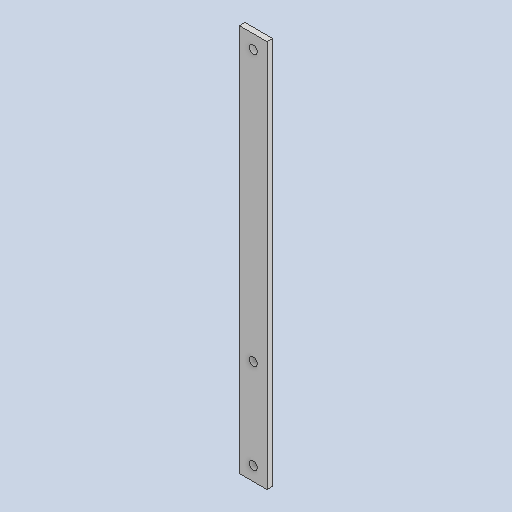
# Autodesk Inventor part: レール接続
Saved by Autodesk Inventor 2022 (Build 260153070, 153G)
## iProperties
Created: 2022-10-17
Part Number: レール接続
Material: 一般
Document SubType Name: Modeling
Designer: hirok
Density: 1 g/cm^3
Appearance: 既定
Author: hirok
Autodesk Inventor part; units mm, degrees
ref_plane "YZ Plane" through (0, 0, 0) normal (1, 0, 0) x (0, 1, 0)
ref_plane "XZ Plane" through (0, 0, 0) normal (0, 1, 0) x (-1, 0, 0)
ref_plane "XY Plane" through (0, 0, 0) normal (0, 0, 1) x (1, 0, 0)
sketch "スケッチ1" plane through (0, 0, 0) normal (0, 0, 1) x (1, 0, 0)
  line L0 (0, 0) -> (10, 0)
  line L1 (10, 0) -> (10, 140)
  line L2 (10, 140) -> (0, 140)
  line L3 (0, 140) -> (0, 0)
  dimension "d0" = 10
  dimension "d1" = 140
  constraints: 8 end point, 2 parallel, 1 horizontal, 1 perpendicular
  measures "d0" distance of L0.start L0.end
  measures "d1" distance of L2.end L0.start
extrude "押し出し1" add sketch "スケッチ1" along normal blind 2
sketch "スケッチ2" plane through (0, 0, 2) normal (0, 0, 1) x (1, 0, 0)
  line L0 (10, 0) -> (10, 140) projected
  line L1 (0, 0) -> (10, 0) projected
  line L2 (10, 140) -> (0, 140) projected
  point P0 (5, 5)
  point P1 (5, 135)
  dimension "d4" = 5
  dimension "d5" = 5
  dimension "d6" = 5
  dimension "d7" = 5
  measures "d4" distance from line of L0 point (5, 135)
  measures "d5" distance from line of L0 point (5, 5)
  measures "d6" distance from line of L1 point (5, 5)
  measures "d7" distance from line of L2 point (5, 135)
hole "穴1" at (5, 5, 2) at (5, 135, 2) direction (0, 0, -1) diameter 3 end through all
sketch "スケッチ3" plane through (0, 0, 2) normal (0, 0, 1) x (1, 0, 0)
  circle A0 centre (5, 5) radius 1.5 projected
  point P0 (0, 0)
  point P1 (5, 37.5)
  dimension "d15" = 32.5
  measures "d15" distance of A0.centre point (5, 37.5)
hole "穴2" at (5, 37.5, 2) direction (0, 0, -1) diameter 3 end through all
